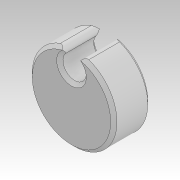
# Autodesk Inventor part: CamShaft
Saved by Autodesk Inventor 2020 (Build 240168000, 168)
## iProperties
Created: 2022-02-03
Part Number: CamShaft
Material: Generic
Document SubType Name: Modeling
Designer: DDeGo
Density: 1 g/cm^3
Appearance: Default
Author: DDeGo
Autodesk Inventor part; units mm, degrees
ref_plane "YZ Plane" through (0, 0, 0) normal (1, 0, 0) x (0, 1, 0)
ref_plane "XZ Plane" through (0, 0, 0) normal (0, 1, 0) x (-1, 0, 0)
ref_plane "XY Plane" through (0, 0, 0) normal (0, 0, 1) x (1, 0, 0)
sketch "Sketch1" plane through (0, 0, 0) normal (0, 0, 1) x (1, 0, 0)
  circle A0 centre (0, 0) radius 4
  dimension "d0" = 8
  constraints: 1 centre point, 1 coincident
  measures "d0" diameter of A0
extrude "Extrusion1" add sketch "Sketch1" along normal blind 3.5
sketch "Sketch4" plane through (0, 0, 0) normal (0, 0, -1) x (-1, 0, 0)
  line L0 (0, 0) -> (0, 2.5)
  circle A0 centre (0, 2.5) radius 1.1
  dimension "d9" = 2.5
  dimension "d10" = 2.2
  constraints: 2 end point, 1 centre point, 1 coincident, 1 vertical
  measures "d9" distance of L0.start L0.end
  measures "d10" diameter of A0
extrude "Extrusion3" cut sketch "Sketch4" against normal through all
chamfer "Chamfer1" distance 0.3 angle 45 4 edges at (-4, 0, 3.5) (-4, 0, 0) (1.1, 2.5, 0) (1.1, 2.5, 3.5)
sketch "Sketch5" plane through (0, 0, 3.5) normal (0, 0, 1) x (1, 0, 0)
  line L0 (-0.4, 4.2659) -> (0.4, 4.2659)
  line L1 (0.4, 4.2659) -> (0.4, 2.9071)
  line L2 (0.4, 2.9071) -> (-0.4, 2.9071)
  line L3 (-0.4, 2.9071) -> (-0.4, 4.2659)
  circle A0 centre (0, 2.5) radius 1.1 construction
  point P0 (0, 0)
  dimension "d16" = 0.4
  dimension "d17" = 0.4
  constraints: 8 end point, 2 parallel, 1 horizontal, 1 perpendicular
  measures "d16" distance from line of L1 A0.centre
  measures "d17" distance from line of A0.centre L3
extrude "Extrusion4" cut sketch "Sketch5" against normal through all
fillet "Fillet1" radius 0.4 4 edges at (-0.4, 3.5247, 1.75) (-0.4, 3.9799, 1.75) (0.4, 3.5247, 1.75) (0.4, 3.9799, 1.75)
equation "\"d17\" = d16"
body "Solid1"
